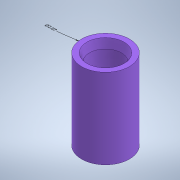
# Autodesk Inventor part: BaseForSvBonyPlosse-40mm
Saved by Autodesk Inventor 2021.1 (Build 251245010, 245A)
## iProperties
Created: 2020-10-08
Part Number: BaseForSvBonyPlosse-40mm
Material: PC/ABS Plastic
Document SubType Name: Modeling
Designer: robst
Density: 0.357273 g/cm^3
Appearance: Violet
Author: robst
Autodesk Inventor part; units mm, degrees
ref_plane "YZ Plane" through (0, 0, 0) normal (1, 0, 0) x (0, 1, 0)
ref_plane "XZ Plane" through (0, 0, 0) normal (0, 1, 0) x (-1, 0, 0)
ref_plane "XY Plane" through (0, 0, 0) normal (0, 0, 1) x (1, 0, 0)
sketch "Sketch1" plane through (0, 0, 0) normal (0, 0, 1) x (1, 0, 0)
  line L0 (0, 0) -> (0, 15.8591) construction
  line L1 (16.51, 0) -> (16.51, 25.4)
  line L2 (16.51, 25.4) -> (17.399, 25.4)
  line L3 (17.399, 25.4) -> (17.399, 43.942)
  line L4 (17.399, 43.942) -> (17.653, 43.942)
  line L5 (17.653, 43.942) -> (17.653, 74.676)
  line L6 (17.653, 74.676) -> (20.447, 83.566)
  line L7 (24.257, 0) -> (16.51, 0)
  line L8 (0, -4.7625) -> (0, 0)
  line L9 (0, 0) -> (16.51, 0)
  line L10 (0, 0) -> (13.335, 0)
  line L11 (13.335, 0) -> (13.335, 15.24)
  line L12 (13.335, 15.24) -> (0, 15.24)
  line L13 (0, 15.24) -> (0, 0)
  line L14 (20.447, 83.566) -> (21.5811, 83.566)
  line L15 (21.5811, 83.566) -> (21.5811, 96.266)
  line L16 (21.5811, 96.266) -> (26.3436, 96.266)
  line L17 (0, -4.7625) -> (26.3436, -4.7625)
  line L18 (26.3436, 96.266) -> (26.3436, -4.7625)
  dimension "d0" = 16.51
  dimension "d1" = 25.4
  dimension "d2" = 17.399
  dimension "d3" = 18.542
  dimension "d4" = 17.653
  dimension "d5" = 30.734
  dimension "d6" = 20.447
  dimension "d14" = 15.24
  dimension "d15" = 3.175
  dimension "d20" = 8.89
  dimension "d23" = 4.7625
  dimension "d24" = 21.5811
  dimension "d25" = 4.7625
  dimension "d82" = 12.7
  constraints: 38 end point, 6 perpendicular, 5 horizontal, 3 vertical, 2 parallel
  measures "d0" distance of L1.start L0.start
  measures "d1" distance of L1.end L1.start
  measures "d2" distance from line of L3 L0.start
  measures "d3" distance of L2.end L3.end
  measures "d4" distance from line of L5 L0.start
  measures "d5" distance of L4.end L5.end
  measures "d6" horizontal distance of L6.end L0.start
  measures "d14" distance from line of L12 L0.start
  measures "d15" distance between parallel lines of L11 L1
  measures "d20" vertical distance of L5.end L6.end
  measures "d23" distance of L15.end L16.end
  measures "d24" distance from line of L15 L0.start
  measures "d25" distance of L8.start L0.start
  measures "d82" distance from line of L14.end L16
revolve "Revolution2" add sketch "Sketch1" angle 360 about axis through (0, 0, 0) along (0, 1, 0)
sketch "Sketch3" plane through (0, -4.7625, 0) normal (0, -1, 0) x (1, 0, 0)
  circle A0 centre (0, 0) radius 19.7577 construction
  line L0 (-18.3966, 4.8114) -> (-18.5034, 4.0625)
  line L1 (-18.5034, 4.0625) -> (-16.3434, 3.7545)
  line L2 (-16.3434, 3.7545) -> (-16.4589, 2.9445)
  line L3 (-16.4589, 2.9445) -> (-18.6189, 3.2525)
  line L4 (-18.6189, 3.2525) -> (-19.0147, 0.4761)
  line L5 (-19.0147, 0.4761) -> (-19.9012, 0.6025)
  line L6 (-19.9012, 0.6025) -> (-22.7402, 3.8765)
  line L7 (-22.7402, 3.8765) -> (-22.6298, 4.6509)
  line L8 (-22.6298, 4.6509) -> (-19.1809, 4.1591)
  line L9 (-19.1809, 4.1591) -> (-19.0741, 4.908)
  line L10 (-19.0741, 4.908) -> (-18.3966, 4.8114)
  line L11 (-19.2964, 3.3491) -> (-21.7519, 3.6992)
  line L12 (-21.7519, 3.6992) -> (-19.5979, 1.235)
  line L13 (-19.5979, 1.235) -> (-19.2964, 3.3491)
  spline S0 degree 2 poles (-17.2788, 10.0487) (-15.7223, 9.3445) (-14.6736, 7.7799) (-15.0999, 6.8376) knots 0 0 0 1 2 2 2
  spline S1 degree 2 poles (-15.0999, 6.8376) (-15.5327, 5.8812) (-17.424, 5.6581) (-18.9477, 6.3475) knots 0 0 0 1 2 2 2
  spline S2 degree 2 poles (-18.9477, 6.3475) (-20.5136, 7.056) (-21.5529, 8.6163) (-21.1244, 9.5634) knots 0 0 0 1 2 2 2
  spline S3 degree 2 poles (-21.1244, 9.5634) (-20.6938, 10.5151) (-18.7884, 10.7318) (-17.2788, 10.0487) knots 0 0 0 1 2 2 2
  spline S4 degree 2 poles (-15.9657, 8.2572) (-16.2007, 8.4991) (-17.0397, 8.9917) (-17.6351, 9.2611) knots 0 0 0 1 2 2 2
  spline S5 degree 2 poles (-17.6351, 9.2611) (-18.2306, 9.5305) (-19.1497, 9.8334) (-19.4981, 9.8498) knots 0 0 0 1 2 2 2
  spline S6 degree 2 poles (-19.4981, 9.8498) (-19.8465, 9.8663) (-20.3358, 9.5962) (-20.4821, 9.2728) knots 0 0 0 1 2 2 2
  spline S7 degree 2 poles (-20.4821, 9.2728) (-20.6285, 8.9493) (-20.5126, 8.3941) (-20.263, 8.1343) knots 0 0 0 1 2 2 2
  spline S8 degree 2 poles (-20.263, 8.1343) (-20.0206, 7.8835) (-19.1587, 7.3918) (-18.5914, 7.1352) knots 0 0 0 1 2 2 2
  spline S9 degree 2 poles (-18.5914, 7.1352) (-17.9819, 6.8594) (-17.1322, 6.5653) (-16.7582, 6.543) knots 0 0 0 1 2 2 2
  spline S10 degree 2 poles (-16.7582, 6.543) (-16.4073, 6.5197) (-15.895, 6.7906) (-15.7422, 7.1282) knots 0 0 0 1 2 2 2
  spline S11 degree 2 poles (-15.7422, 7.1282) (-15.598, 7.447) (-15.714, 8.0021) (-15.9657, 8.2572) knots 0 0 0 1 2 2 2
  line L14 (-7.9032, 14.904) -> (-9.5179, 17.1401)
  spline S12 degree 2 poles (-9.5179, 17.1401) (-9.7107, 17.4071) (-10.0808, 17.8317) (-10.238, 17.9086) knots 0 0 0 1 2 2 2
  spline S13 degree 2 poles (-10.238, 17.9086) (-10.4041, 17.9981) (-10.755, 17.9478) (-10.9761, 17.7881) knots 0 0 0 1 2 2 2
  spline S14 degree 2 poles (-10.9761, 17.7881) (-11.1764, 17.6435) (-11.4575, 17.066) (-11.5308, 16.6577) knots 0 0 0 1 2 2 2
  spline S15 degree 2 poles (-11.5308, 16.6577) (-11.4844, 16.6023) (-11.3586, 16.4456) (-11.2803, 16.3371) knots 0 0 0 1 2 2 2
  line L15 (-11.2803, 16.3371) -> (-9.4426, 13.7923)
  line L16 (-9.4426, 13.7923) -> (-10.0934, 13.3223)
  line L17 (-10.0934, 13.3223) -> (-11.7081, 15.5584)
  spline S16 degree 2 poles (-11.7081, 15.5584) (-11.901, 15.8254) (-12.271, 16.25) (-12.4282, 16.327) knots 0 0 0 1 2 2 2
  spline S17 degree 2 poles (-12.4282, 16.327) (-12.5943, 16.4165) (-12.9452, 16.3662) (-13.1663, 16.2065) knots 0 0 0 1 2 2 2
  spline S18 degree 2 poles (-13.1663, 16.2065) (-13.3749, 16.0559) (-13.6482, 15.4587) (-13.7175, 15.0976) knots 0 0 0 1 2 2 2
  line L18 (-13.7175, 15.0976) -> (-11.6328, 12.2107)
  line L19 (-11.6328, 12.2107) -> (-12.2836, 11.7407)
  line L20 (-12.2836, 11.7407) -> (-15.0733, 15.6038)
  line L21 (-15.0733, 15.6038) -> (-14.4225, 16.0738)
  line L22 (-14.4225, 16.0738) -> (-14.1152, 15.6483)
  spline S19 degree 2 poles (-14.1152, 15.6483) (-14.0445, 16.0865) (-13.7457, 16.7275) (-13.4453, 16.9445) knots 0 0 0 1 2 2 2
  spline S20 degree 2 poles (-13.4453, 16.9445) (-13.1032, 17.1915) (-12.3475, 17.2612) (-11.9537, 17.006) knots 0 0 0 1 2 2 2
  spline S21 degree 2 poles (-11.9537, 17.006) (-11.8955, 17.5495) (-11.5805, 18.2911) (-11.2551, 18.5261) knots 0 0 0 1 2 2 2
  spline S22 degree 2 poles (-11.2551, 18.5261) (-11.0048, 18.7068) (-10.4845, 18.8477) (-10.2078, 18.781) knots 0 0 0 1 2 2 2
  spline S23 degree 2 poles (-10.2078, 18.781) (-9.9269, 18.7172) (-9.3763, 18.3151) (-9.0901, 17.9187) knots 0 0 0 1 2 2 2
  line L23 (-9.0901, 17.9187) -> (-7.2524, 15.3739)
  line L24 (-7.2524, 15.3739) -> (-7.9032, 14.904)
  line L25 (-0.9371, 16.8437) -> (-1.4673, 19.5504)
  spline S24 degree 2 poles (-1.4673, 19.5504) (-1.5306, 19.8736) (-1.689, 20.4142) (-1.7994, 20.5499) knots 0 0 0 1 2 2 2
  spline S25 degree 2 poles (-1.7994, 20.5499) (-1.9129, 20.7007) (-2.2526, 20.8019) (-2.5202, 20.7495) knots 0 0 0 1 2 2 2
  spline S26 degree 2 poles (-2.5202, 20.7495) (-2.7626, 20.702) (-3.2597, 20.2953) (-3.4972, 19.9551) knots 0 0 0 1 2 2 2
  spline S27 degree 2 poles (-3.4972, 19.9551) (-3.4783, 19.8854) (-3.4297, 19.6904) (-3.4039, 19.5591) knots 0 0 0 1 2 2 2
  line L26 (-3.4039, 19.5591) -> (-2.8005, 16.4787)
  line L27 (-2.8005, 16.4787) -> (-3.5883, 16.3244)
  line L28 (-3.5883, 16.3244) -> (-4.1185, 19.0311)
  spline S28 degree 2 poles (-4.1185, 19.0311) (-4.1818, 19.3543) (-4.3402, 19.8949) (-4.4506, 20.0305) knots 0 0 0 1 2 2 2
  spline S29 degree 2 poles (-4.4506, 20.0305) (-4.5641, 20.1813) (-4.9038, 20.2826) (-5.1714, 20.2302) knots 0 0 0 1 2 2 2
  spline S30 degree 2 poles (-5.1714, 20.2302) (-5.4239, 20.1807) (-5.9221, 19.7528) (-6.1363, 19.4539) knots 0 0 0 1 2 2 2
  line L29 (-6.1363, 19.4539) -> (-5.4517, 15.9594)
  line L30 (-5.4517, 15.9594) -> (-6.2395, 15.805)
  line L31 (-6.2395, 15.805) -> (-7.1555, 20.4813)
  line L32 (-7.1555, 20.4813) -> (-6.3677, 20.6356)
  line L33 (-6.3677, 20.6356) -> (-6.2668, 20.1205)
  spline S31 degree 2 poles (-6.2668, 20.1205) (-6.0191, 20.4889) (-5.4794, 20.9459) (-5.1158, 21.0171) knots 0 0 0 1 2 2 2
  spline S32 degree 2 poles (-5.1158, 21.0171) (-4.7017, 21.0982) (-3.9862, 20.8451) (-3.7355, 20.4485) knots 0 0 0 1 2 2 2
  spline S33 degree 2 poles (-3.7355, 20.4485) (-3.4551, 20.9177) (-2.8585, 21.4593) (-2.4646, 21.5365) knots 0 0 0 1 2 2 2
  spline S34 degree 2 poles (-2.4646, 21.5365) (-2.1616, 21.5958) (-1.6301, 21.5059) (-1.4068, 21.3294) knots 0 0 0 1 2 2 2
  spline S35 degree 2 poles (-1.4068, 21.3294) (-1.1784, 21.1539) (-0.8467, 20.5582) (-0.7528, 20.0785) knots 0 0 0 1 2 2 2
  line L34 (-0.7528, 20.0785) -> (-0.1493, 16.998)
  line L35 (-0.1493, 16.998) -> (-0.9371, 16.8437)
  spline S36 degree 2 poles (6.024, 15.4728) (5.4421, 15.6793) (4.5971, 16.4215) (4.3776, 16.9417) knots 0 0 0 1 2 2 2
  spline S37 degree 2 poles (4.3776, 16.9417) (4.1564, 17.457) (4.1767, 18.7603) (4.4452, 19.5168) knots 0 0 0 1 2 2 2
  spline S38 degree 2 poles (4.4452, 19.5168) (4.712, 20.2685) (5.491, 21.2479) (6.001, 21.531) knots 0 0 0 1 2 2 2
  spline S39 degree 2 poles (6.001, 21.531) (6.5027, 21.8062) (7.6321, 21.8804) (8.2382, 21.6652) knots 0 0 0 1 2 2 2
  spline S40 degree 2 poles (8.2382, 21.6652) (8.5389, 21.5585) (9.0365, 21.2836) (9.2355, 21.1366) knots 0 0 0 1 2 2 2
  spline S41 degree 2 poles (9.2355, 21.1366) (9.4071, 21.0047) (9.7459, 20.6824) (9.9069, 20.5051) knots 0 0 0 1 2 2 2
  line L36 (9.9069, 20.5051) -> (9.5661, 19.5449)
  line L37 (9.5661, 19.5449) -> (9.5031, 19.5673)
  spline S42 degree 2 poles (9.5031, 19.5673) (9.4308, 19.7022) (9.1974, 20.0908) (9.0063, 20.306) knots 0 0 0 1 2 2 2
  spline S43 degree 2 poles (9.0063, 20.306) (8.8231, 20.513) (8.3416, 20.8641) (7.9924, 20.988) knots 0 0 0 1 2 2 2
  spline S44 degree 2 poles (7.9924, 20.988) (7.6093, 21.124) (6.8137, 21.0515) (6.4499, 20.842) knots 0 0 0 1 2 2 2
  spline S45 degree 2 poles (6.4499, 20.842) (6.0893, 20.626) (5.4793, 19.7996) (5.2745, 19.2225) knots 0 0 0 1 2 2 2
  spline S46 degree 2 poles (5.2745, 19.2225) (5.0559, 18.6066) (5.0367, 17.6142) (5.1853, 17.2174) knots 0 0 0 1 2 2 2
  spline S47 degree 2 poles (5.1853, 17.2174) (5.3325, 16.8321) (5.8999, 16.2922) (6.2781, 16.158) knots 0 0 0 1 2 2 2
  spline S48 degree 2 poles (6.2781, 16.158) (6.6224, 16.0358) (7.2695, 15.9972) (7.5421, 16.0424) knots 0 0 0 1 2 2 2
  spline S49 degree 2 poles (7.5421, 16.0424) (7.8051, 16.091) (8.223, 16.2376) (8.3478, 16.297) knots 0 0 0 1 2 2 2
  line L38 (8.3478, 16.297) -> (8.406, 16.2764)
  line L39 (8.406, 16.2764) -> (8.0687, 15.3259)
  spline S50 degree 2 poles (8.0687, 15.3259) (7.8371, 15.3043) (7.4277, 15.2585) (7.1529, 15.2687) knots 0 0 0 1 2 2 2
  spline S51 degree 2 poles (7.1529, 15.2687) (6.86, 15.2743) (6.3829, 15.3454) (6.024, 15.4728) knots 0 0 0 1 2 2 2
  spline S52 degree 2 poles (10.945, 13.32) (10.8235, 13.3197) (10.4058, 13.3071) (10.2357, 13.3362) knots 0 0 0 1 2 2 2
  spline S53 degree 2 poles (10.2357, 13.3362) (9.9986, 13.3697) (9.6091, 13.5087) (9.3187, 13.7218) knots 0 0 0 1 2 2 2
  spline S54 degree 2 poles (9.3187, 13.7218) (9.0822, 13.8953) (8.7858, 14.3873) (8.7427, 14.6678) knots 0 0 0 1 2 2 2
  spline S55 degree 2 poles (8.7427, 14.6678) (8.7049, 14.9381) (8.8591, 15.5398) (9.0479, 15.797) knots 0 0 0 1 2 2 2
  spline S56 degree 2 poles (9.0479, 15.797) (9.3401, 16.1953) (10.0902, 16.5129) (10.574, 16.4068) knots 0 0 0 1 2 2 2
  spline S57 degree 2 poles (10.574, 16.4068) (11.0072, 16.3188) (11.969, 15.7854) (12.5006, 15.44) knots 0 0 0 1 2 2 2
  line L40 (12.5006, 15.44) -> (12.5919, 15.5645)
  spline S58 degree 2 poles (12.5919, 15.5645) (12.7563, 15.7885) (12.8234, 16.1669) (12.7567, 16.3371) knots 0 0 0 1 2 2 2
  spline S59 degree 2 poles (12.7567, 16.3371) (12.6901, 16.5072) (12.3698, 16.8188) (12.179, 16.9589) knots 0 0 0 1 2 2 2
  spline S60 degree 2 poles (12.179, 16.9589) (11.955, 17.1232) (11.2518, 17.4349) (10.8546, 17.5286) knots 0 0 0 1 2 2 2
  line L41 (10.8546, 17.5286) -> (10.8172, 17.556)
  line L42 (10.8172, 17.556) -> (11.3013, 18.2156)
  spline S61 degree 2 poles (11.3013, 18.2156) (11.5162, 18.1345) (12.2755, 17.7688) (12.6033, 17.5283) knots 0 0 0 1 2 2 2
  spline S62 degree 2 poles (12.6033, 17.5283) (13.0015, 17.2361) (13.4537, 16.7128) (13.5507, 16.3927) knots 0 0 0 1 2 2 2
  spline S63 degree 2 poles (13.5507, 16.3927) (13.6466, 16.0798) (13.4857, 15.4256) (13.2209, 15.0647) knots 0 0 0 1 2 2 2
  line L43 (13.2209, 15.0647) -> (11.2938, 12.4385)
  line L44 (11.2938, 12.4385) -> (10.6466, 12.9134)
  line L45 (10.6466, 12.9134) -> (10.945, 13.32)
  line L46 (11.3407, 13.8593) -> (12.1231, 14.9255)
  spline S64 degree 2 poles (12.1231, 14.9255) (11.8755, 15.0753) (11.1226, 15.5192) (10.854, 15.6142) knots 0 0 0 1 2 2 2
  spline S65 degree 2 poles (10.854, 15.6142) (10.539, 15.7241) (9.9624, 15.6429) (9.7493, 15.3525) knots 0 0 0 1 2 2 2
  spline S66 degree 2 poles (9.7493, 15.3525) (9.5058, 15.0206) (9.6326, 14.4106) (9.9894, 14.1488) knots 0 0 0 1 2 2 2
  spline S67 degree 2 poles (9.9894, 14.1488) (10.2923, 13.9265) (10.9819, 13.8226) (11.3407, 13.8593) knots 0 0 0 1 2 2 2
  spline S68 degree 2 poles (12.7981, 10.5668) (12.4952, 10.9373) (12.17, 11.7416) (12.1089, 12.0439) knots 0 0 0 1 2 2 2
  line L47 (12.1089, 12.0439) -> (12.8061, 12.6139)
  line L48 (12.8061, 12.6139) -> (12.8321, 12.5821)
  spline S69 degree 2 poles (12.8321, 12.5821) (12.8335, 12.4503) (12.858, 12.1114) (12.921, 11.8637) knots 0 0 0 1 2 2 2
  spline S70 degree 2 poles (12.921, 11.8637) (12.9723, 11.6464) (13.1734, 11.1728) (13.3396, 10.9696) knots 0 0 0 1 2 2 2
  spline S71 degree 2 poles (13.3396, 10.9696) (13.4601, 10.8222) (13.8047, 10.539) (13.9256, 10.5049) knots 0 0 0 1 2 2 2
  spline S72 degree 2 poles (13.9256, 10.5049) (14.0957, 10.4512) (14.3517, 10.4877) (14.527, 10.631) knots 0 0 0 1 2 2 2
  spline S73 degree 2 poles (14.527, 10.631) (14.7461, 10.8102) (14.7778, 11.2349) (14.6027, 11.6035) knots 0 0 0 1 2 2 2
  spline S74 degree 2 poles (14.6027, 11.6035) (14.5328, 11.7458) (14.2998, 12.1934) (14.2101, 12.3926) knots 0 0 0 1 2 2 2
  spline S75 degree 2 poles (14.2101, 12.3926) (13.9883, 12.9158) (14.1856, 13.7152) (14.5481, 14.0116) knots 0 0 0 1 2 2 2
  spline S76 degree 2 poles (14.5481, 14.0116) (15.05, 14.422) (16.2911, 14.1804) (16.7992, 13.559) knots 0 0 0 1 2 2 2
  spline S77 degree 2 poles (16.7992, 13.559) (17.05, 13.2522) (17.4068, 12.507) (17.4639, 12.2014) knots 0 0 0 1 2 2 2
  line L49 (17.4639, 12.2014) -> (16.7986, 11.6574)
  line L50 (16.7986, 11.6574) -> (16.7725, 11.6893)
  spline S78 degree 2 poles (16.7725, 11.6893) (16.7683, 12.0847) (16.5119, 12.8454) (16.2676, 13.1442) knots 0 0 0 1 2 2 2
  spline S79 degree 2 poles (16.2676, 13.1442) (16.0168, 13.451) (15.4126, 13.6616) (15.1536, 13.4498) knots 0 0 0 1 2 2 2
  spline S80 degree 2 poles (15.1536, 13.4498) (14.9186, 13.2577) (14.8967, 12.821) (15.053, 12.4835) knots 0 0 0 1 2 2 2
  spline S81 degree 2 poles (15.053, 12.4835) (15.1279, 12.3188) (15.3363, 11.9175) (15.4456, 11.6945) knots 0 0 0 1 2 2 2
  spline S82 degree 2 poles (15.4456, 11.6945) (15.6742, 11.2034) (15.5389, 10.4015) (15.1286, 10.066) knots 0 0 0 1 2 2 2
  spline S83 degree 2 poles (15.1286, 10.066) (14.8895, 9.8706) (14.3142, 9.7126) (14.009, 9.7688) knots 0 0 0 1 2 2 2
  spline S84 degree 2 poles (14.009, 9.7688) (13.686, 9.8304) (13.1076, 10.1884) (12.7981, 10.5668) knots 0 0 0 1 2 2 2
  spline S85 degree 2 poles (15.2194, 6.6414) (14.7404, 7.6785) (15.3771, 9.3557) (16.4516, 9.852) knots 0 0 0 1 2 2 2
  spline S86 degree 2 poles (16.4516, 9.852) (17.5074, 10.3396) (19.2707, 9.8108) (19.6829, 8.9185) knots 0 0 0 1 2 2 2
  spline S87 degree 2 poles (19.6829, 8.9185) (19.8684, 8.5167) (19.9219, 7.7875) (19.78, 7.4442) knots 0 0 0 1 2 2 2
  spline S88 degree 2 poles (19.78, 7.4442) (19.6403, 7.0963) (19.0399, 6.5186) (18.5213, 6.279) knots 0 0 0 1 2 2 2
  line L51 (18.5213, 6.279) -> (18.1243, 6.0956)
  line L52 (18.1243, 6.0956) -> (16.7411, 9.0901)
  spline S89 degree 2 poles (16.7411, 9.0901) (15.989, 8.7427) (15.5397, 7.617) (15.8504, 6.9442) knots 0 0 0 1 2 2 2
  spline S90 degree 2 poles (15.8504, 6.9442) (15.9605, 6.706) (16.2815, 6.2931) (16.4519, 6.1451) knots 0 0 0 1 2 2 2
  spline S91 degree 2 poles (16.4519, 6.1451) (16.636, 5.9921) (16.9247, 5.7966) (17.0404, 5.7424) knots 0 0 0 1 2 2 2
  line L53 (17.0404, 5.7424) -> (17.0598, 5.7003)
  line L54 (17.0598, 5.7003) -> (16.2656, 5.3335)
  spline S92 degree 2 poles (16.2656, 5.3335) (16.156, 5.4359) (15.8296, 5.7499) (15.7185, 5.88) knots 0 0 0 1 2 2 2
  spline S93 degree 2 poles (15.7185, 5.88) (15.5606, 6.0622) (15.3402, 6.3798) (15.2194, 6.6414) knots 0 0 0 1 2 2 2
  spline S94 degree 2 poles (18.3522, 7.0625) (18.6422, 7.2078) (19.0159, 7.5278) (19.1067, 7.7114) knots 0 0 0 1 2 2 2
  spline S95 degree 2 poles (19.1067, 7.7114) (19.212, 7.9131) (19.2014, 8.39) (19.0655, 8.6843) knots 0 0 0 1 2 2 2
  spline S96 degree 2 poles (19.0655, 8.6843) (18.9317, 8.974) (18.5711, 9.3006) (18.3253, 9.3911) knots 0 0 0 1 2 2 2
  spline S97 degree 2 poles (18.3253, 9.3911) (18.0769, 9.4747) (17.5835, 9.4509) (17.297, 9.3469) knots 0 0 0 1 2 2 2
  line L55 (17.297, 9.3469) -> (18.3522, 7.0625)
  line L56 (22.9917, -3.1507) -> (16.6951, -0.8142)
  line L57 (16.6951, -0.8142) -> (16.7167, 0.0963)
  line L58 (16.7167, 0.0963) -> (23.1166, 2.1326)
  line L59 (23.1166, 2.1326) -> (23.0952, 1.2272)
  line L60 (23.0952, 1.2272) -> (17.7805, -0.4075)
  line L61 (17.7805, -0.4075) -> (23.012, -2.2916)
  line L62 (23.012, -2.2916) -> (22.9917, -3.1507)
  spline S98 degree 2 poles (18.2186, -8.2229) (16.598, -7.6821) (15.3944, -6.2334) (15.7218, -5.2522) knots 0 0 0 1 2 2 2
  spline S99 degree 2 poles (15.7218, -5.2522) (16.0541, -4.2565) (17.9126, -3.8406) (19.499, -4.37) knots 0 0 0 1 2 2 2
  spline S100 degree 2 poles (19.499, -4.37) (21.1293, -4.9141) (22.3232, -6.3595) (21.9942, -7.3455) knots 0 0 0 1 2 2 2
  spline S101 degree 2 poles (21.9942, -7.3455) (21.6635, -8.3364) (19.7903, -8.7474) (18.2186, -8.2229) knots 0 0 0 1 2 2 2
  spline S102 degree 2 poles (16.7286, -6.5756) (16.9873, -6.7921) (17.8724, -7.196) (18.4923, -7.4028) knots 0 0 0 1 2 2 2
  spline S103 degree 2 poles (18.4923, -7.4028) (19.1122, -7.6097) (20.0576, -7.8167) (20.4058, -7.7973) knots 0 0 0 1 2 2 2
  spline S104 degree 2 poles (20.4058, -7.7973) (20.754, -7.7779) (21.213, -7.4591) (21.3254, -7.1223) knots 0 0 0 1 2 2 2
  spline S105 degree 2 poles (21.3254, -7.1223) (21.4378, -6.7855) (21.2655, -6.2452) (20.9906, -6.0124) knots 0 0 0 1 2 2 2
  spline S106 degree 2 poles (20.9906, -6.0124) (20.7238, -5.7878) (19.816, -5.3871) (19.2253, -5.19) knots 0 0 0 1 2 2 2
  spline S107 degree 2 poles (19.2253, -5.19) (18.5908, -4.9783) (17.7154, -4.7729) (17.3411, -4.789) knots 0 0 0 1 2 2 2
  spline S108 degree 2 poles (17.3411, -4.789) (16.9896, -4.8019) (16.5078, -5.124) (16.3905, -5.4754) knots 0 0 0 1 2 2 2
  spline S109 degree 2 poles (16.3905, -5.4754) (16.2798, -5.8073) (16.4521, -6.3476) (16.7286, -6.5756) knots 0 0 0 1 2 2 2
  spline S110 degree 2 poles (18.5839, -12.6105) (18.7157, -12.4201) (18.8832, -11.9791) (18.9372, -11.7474) knots 0 0 0 1 2 2 2
  spline S111 degree 2 poles (18.9372, -11.7474) (18.9824, -11.5283) (19.0029, -11.1733) (19.0025, -11.0291) knots 0 0 0 1 2 2 2
  line L63 (19.0025, -11.0291) -> (19.0318, -10.9868)
  line L64 (19.0318, -10.9868) -> (19.7723, -11.4992)
  spline S112 degree 2 poles (19.7723, -11.4992) (19.7369, -11.8126) (19.394, -12.7331) (19.151, -13.0843) knots 0 0 0 1 2 2 2
  spline S113 degree 2 poles (19.151, -13.0843) (18.905, -13.4397) (18.3951, -13.8691) (18.0934, -13.9795) knots 0 0 0 1 2 2 2
  spline S114 degree 2 poles (18.0934, -13.9795) (17.7702, -14.0938) (17.1281, -13.9998) (16.8065, -13.7773) knots 0 0 0 1 2 2 2
  spline S115 degree 2 poles (16.8065, -13.7773) (16.3749, -13.4786) (16.1157, -12.4606) (16.3063, -12.0043) knots 0 0 0 1 2 2 2
  line L65 (16.3063, -12.0043) -> (16.2555, -11.9692)
  spline S116 degree 2 poles (16.2555, -11.9692) (16.1075, -12.1108) (15.6945, -12.3819) (15.4309, -12.4373) knots 0 0 0 1 2 2 2
  spline S117 degree 2 poles (15.4309, -12.4373) (15.1715, -12.4956) (14.5571, -12.3708) (14.2143, -12.1336) knots 0 0 0 1 2 2 2
  spline S118 degree 2 poles (14.2143, -12.1336) (13.8631, -11.8905) (13.4334, -11.2364) (13.3572, -10.8583) knots 0 0 0 1 2 2 2
  spline S119 degree 2 poles (13.3572, -10.8583) (13.2783, -10.4658) (13.4809, -9.6485) (13.765, -9.2381) knots 0 0 0 1 2 2 2
  spline S120 degree 2 poles (13.765, -9.2381) (14.0373, -8.8446) (14.7607, -8.2062) (15.0734, -8.0346) knots 0 0 0 1 2 2 2
  line L66 (15.0734, -8.0346) -> (15.8139, -8.5471)
  line L67 (15.8139, -8.5471) -> (15.7788, -8.5979)
  spline S121 degree 2 poles (15.7788, -8.5979) (15.4657, -8.7066) (14.6541, -9.2464) (14.3994, -9.6145) knots 0 0 0 1 2 2 2
  spline S122 degree 2 poles (14.3994, -9.6145) (14.25, -9.8303) (14.0867, -10.3556) (14.1437, -10.6078) knots 0 0 0 1 2 2 2
  spline S123 degree 2 poles (14.1437, -10.6078) (14.2037, -10.8558) (14.4735, -11.2616) (14.757, -11.4578) knots 0 0 0 1 2 2 2
  spline S124 degree 2 poles (14.757, -11.4578) (15.0405, -11.654) (15.5229, -11.7438) (15.7312, -11.6689) knots 0 0 0 1 2 2 2
  spline S125 degree 2 poles (15.7312, -11.6689) (15.9394, -11.594) (16.298, -11.2476) (16.462, -11.0107) knots 0 0 0 1 2 2 2
  line L68 (16.462, -11.0107) -> (16.667, -10.7145)
  line L69 (16.667, -10.7145) -> (17.2467, -11.1156)
  line L70 (17.2467, -11.1156) -> (17.0856, -11.3484)
  spline S126 degree 2 poles (17.0856, -11.3484) (16.7606, -11.8181) (16.7992, -12.7209) (17.2265, -13.0166) knots 0 0 0 1 2 2 2
  spline S127 degree 2 poles (17.2265, -13.0166) (17.4254, -13.1543) (17.8143, -13.1981) (17.9839, -13.134) knots 0 0 0 1 2 2 2
  spline S128 degree 2 poles (17.9839, -13.134) (18.1635, -13.0643) (18.458, -12.7925) (18.5839, -12.6105) knots 0 0 0 1 2 2 2
  dimension "d27" = 39.5154
  constraints: 1 centre point, 1 coincident, 1 other
  measures "d27" diameter of A0
emboss "Emboss1" sketch "Sketch3" operation cut depth 1.27 direction (0, 1, 0)
sketch "Sketch9" plane through (0, 0, 0) normal (1, 0, 0) x (0, 1, 0)
  line L0 (83.566, 21.5811) -> (96.266, 21.5811) projected
  line L1 (96.266, 21.5811) -> (96.266, -21.5811) projected
  line L2 (0, 0) -> (96.266, 0) construction
  line L3 (96.266, 26.3436) -> (96.266, -26.3436) construction
  line L4 (96.266, 21.5811) -> (95.6171, 20.4572)
  line L5 (95.4191, 20.4572) -> (94.7702, 21.5811)
  arc A0 (95.4191, 20.4572) -> (95.6171, 20.4572) centre (95.5181, 20.5143) ccw
  dimension "d91" = 60
  dimension "d92" = 0.1143
  dimension "d93" = 20.4
  dimension "d94" = 21.5811
  constraints: 6 end point, 2 point on circle, 2 tangent, 1 centre point, 1 equal length, 1 midpoint, 1 point on line
  measures "d91" angle of L5 L4
  measures "d92" radius of A0
  measures "d93" distance edge to line of A0 L2
  measures "d94" distance between parallel lines of L0 L2
coil "Coil5" sketch "Sketch9" operation add axis through (0, 0, 0) along (0, -1, 0) pitch 2.1167 turns 6 hand right
ref_plane "Work Plane1" through (0, 83.566, 0) normal (0, 1, 0) x (1, 0, 0)
split "Split4" plane through (0, 83.566, 0) removes the side toward (0, 1, 0)
equation "\"d0\" = baseRadius"
equation "\"d1\" = baseHeight"
equation "\"d2\" = middleRadius"
equation "\"d3\" = middleHeight"
equation "\"d4\" = middleTopRadius"
equation "\"d5\" = middleTopHeight"
equation "\"d6\" = topHeightRadius"
equation "\"d14\" = baseInteriorHeight"
equation "\"d15\" = baseWallThickness"
equation "\"d20\" = topHeight"
equation "\"d23\" = wallThickness"
equation "\"d24\" = interiorRadius"
equation "\"d25\" = caseBottomThickness"
equation "\"d82\" = caseHeightAboveLens"
equation "\"d27\" = textRingDiameter"
equation "\"d28\" = textDepth"
equation "\"d92\" = b1RootRadius"
equation "\"d93\" = b1MinorRadius"
equation "\"d95\" = pitch"
equation "\"d96\" = caseHeightAboveLens"
equation "\"baseDiameter\" = 33.02"
equation "\"baseRadius\" = 0.5 * baseDiameter"
equation "\"baseHeight\" = 25.4"
equation "\"middleDiameter\" = 34.798"
equation "\"middleRadius\" = 0.5 * middleDiameter"
equation "\"middleTopDiameter\" = 35.306"
equation "\"middleTopRadius\" = 0.5 * middleTopDiameter"
equation "\"middleHeight\" = 18.542"
equation "\"middleTopHeight\" = 30.734"
equation "\"topBaseDiameter\" = 34.798"
equation "\"topHeightDiameter\" = 40.894"
equation "\"topBaseRadius\" = 0.5 * topBaseDiameter"
equation "\"topHeightRadius\" = 0.5 * topHeightDiameter"
equation "\"topHeight\" = 8.89"
equation "\"d9\" = caseBottomThickness"
equation "\"wallThickness\" = 4.7625"
equation "\"caseBottomThickness\" = 4.7625"
equation "\"caseHeightAboveLens\" = 12.7"
equation "\"baseWallThickness\" = 3.175"
equation "\"baseInteriorHeight\" = 15.24"
equation "\"interiorDiameter\" = b1MajorDiameter"
equation "\"interiorRadius\" = 0.5 * interiorDiameter"
equation "\"outsideRadius\" = interiorRadius + wallThickness"
equation "\"outsideDiameter\" = 2 * outsideRadius"
equation "\"textRingDiameter\" = 0.75 * outsideDiameter"
equation "\"textDepth\" = 1.27"
equation "\"b1MajorDiameter\" = 43.16222"
equation "\"b1MajorRadius\" = 0.5 * b1MajorDiameter"
equation "\"b1MinorDiameter\" = 40.80002"
equation "\"b1MinorRadius\" = 0.5 * b1MinorDiameter"
equation "\"b1RootRadius\" = 0.1143"
equation "\"pitch\" = 2.116667"
body "Solid2"
